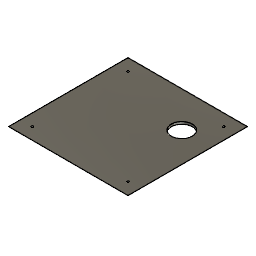
Bloc Bras Gauche 200x200 (Autodesk Fusion 360 design; units mm, degrees)
part number: 2026-03-31-14-11-04-905
Autodesk Fusion 360 part; units mm, degrees
sketch "Esquisse1" plane through (0, 0, 0) normal (0, 0, 1) x (1, 0, 0)
  line L0 (0, 0) -> (200, 0)
  line L1 (200, 0) -> (200, 200)
  line L2 (200, 200) -> (0, 200)
  line L3 (0, 200) -> (0, 0)
  dimension "d18" = 200
  dimension "d19" = 200
  constraint horizontal L0
  constraint vertical L1
  constraint horizontal L2
  constraint vertical L3
  constraint coincident L0.start L3.end
  measures "d18" distance of L0 L2
  measures "d19" distance of L1 L3
extrude "Extrusion1" add sketch "Esquisse1" along normal blind 4
chamfer "Chanfrein1" distance 4 angle 45 1 faces at (66.6667, 133.3333, 0)
sketch "Esquisse2" plane through (0, 0, 4) normal (0, 0, 1) x (-1, 0, 0)
  circle A0 centre (-20, -180) radius 1.5
  circle A1 centre (-180, -180) radius 1.5
  circle A2 centre (-180, -20) radius 1.5
  circle A3 centre (-20, -20) radius 1.5
  line L0 (0, 0) -> (-20, -20)
  line L1 (-200, 0) -> (-180, -20)
  line L2 (-200, 0) -> (-297.1716, 0) construction
  line L3 (0, -200) -> (-20, -180)
  line L4 (-200, -200) -> (-180, -180)
  line L5 (-200, -200) -> (-297.1716, -200) construction
  line L6 (0, -200) -> (0, 0)
  line L7 (0, 0) -> (-200, 0)
  line L8 (-200, 0) -> (-200, -200)
  line L9 (-200, -200) -> (0, -200)
  dimension "d10" = 3
  dimension "d11" = 3
  dimension "d12" = 3
  dimension "d13" = 3
  dimension "d20" = 28.2843
  dimension "d22" = 45
  dimension "d23" = 28.2843
  dimension "d24" = 28.2843
  dimension "d25" = 28.2843
  dimension "d26" = 45
  constraint coincident A3.centre L0.end
  constraint horizontal L2
  constraint coincident A2.centre L1.end
  constraint coincident A0.centre L3.end
  constraint horizontal L5
  constraint coincident A1.centre L4.end
  constraint coincident L1.start L2.start
  constraint coincident L4.start L5.start
  measures "d10" diameter of A0
  measures "d11" diameter of A1
  measures "d12" diameter of A2
  measures "d13" diameter of A3
  measures "d20" distance of L0.start A3.centre
  measures "d22" angle of L1 L2
  measures "d23" distance of A2.centre L1.start
  measures "d24" distance of L3.start A0.centre
  measures "d25" distance of A1.centre L4.start
  measures "d26" angle of L4 L5
extrude "Extrusion2" cut sketch "Esquisse2" against normal blind 14 contours A0 | A1 | A2 | A3
thread "Filetage1" "ISO Metric profile 4.0 M4x0.7 M4x0.7 6H" major diameter 4.1095 minor diameter 3.332 pitch 0.7 angle 60 resizes the face on face at (21.4536, 179.6299, 2.6667)
thread "Filetage2" "ISO Metric profile 4.0 M4x0.7 M4x0.7 6H" major diameter 4.1095 minor diameter 3.332 pitch 0.7 angle 60 resizes the face on face at (21.4925, 20.1494, 1.3333)
thread "Filetage3" "ISO Metric profile 4.0 M4x0.7 M4x0.7 6H" major diameter 4.1095 minor diameter 3.332 pitch 0.7 angle 60 resizes the face on face at (179.3157, 18.6652, 2.6667)
thread "Filetage4" "ISO Metric profile 4.0 M4x0.7 M4x0.7 6H" major diameter 4.1095 minor diameter 3.332 pitch 0.7 angle 60 resizes the face on face at (179.1244, 178.7821, 1.3333)
sketch "Esquisse3" plane through (0, 0, 4) normal (0, 0, 1) x (-1, 0, 0)
  circle A0 centre (-180, -180) radius 1.666
  circle A1 centre (-180, -20) radius 1.666
  circle A2 centre (-20, -180) radius 1.666
  circle A3 centre (-20, -20) radius 1.666
  line L0 (0, -200) -> (0, 0)
  line L1 (0, 0) -> (-200, 0)
  line L2 (-200, 0) -> (-200, -200)
  line L3 (-200, -200) -> (0, -200)
  circle A4 centre (-150, -140) radius 17.5
  point P0 (-150, -140)
  dimension "d28" = 60
  dimension "d29" = 50
  dimension "d30" = 35
  constraint coincident P0 A4.centre
  measures "d28" distance of L3 P0
  measures "d29" distance of L2 P0
  measures "d30" diameter of A4
extrude "Extrusion3" cut sketch "Esquisse3" against normal blind 10 contours A4
equation "d20 = ( sqrt(800) ) * 1 mm"
equation "d23 = ( sqrt(800) ) * 1 mm"
equation "d24 = ( sqrt(800) ) * 1 mm"
equation "d25 = ( sqrt(800) ) * 1 mm"
